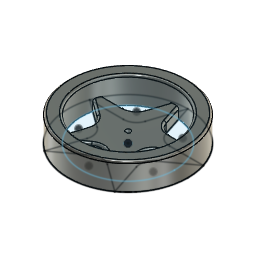
wheel (Autodesk Fusion 360 design; units mm, degrees)
Autodesk Fusion 360 part; units mm, degrees
note: some values were not read from the file. Set by a fixed rule: which sketch regions a step uses.
sketch "Esboço1" plane through (0, 0, 0) normal (0, 0, 1) x (1, 0, 0)
  circle A0 centre (0, 0) radius 45
  circle A1 centre (0, 0) radius 2
  circle A2 centre (0, 0) radius 35
  line L0 (-7.858, 20.8156) -> (0, 45)
  line L1 (-42.7975, 13.9058) -> (-17.3686, 13.9058)
  arc A3 (-17.3686, 13.9058) -> (-7.858, 20.8156) centre (-17.3686, 23.9058) ccw
  line L2 (0, 45) -> (7.858, 20.8156)
  line L3 (42.7975, 13.9058) -> (17.3686, 13.9058)
  arc A4 (7.858, 20.8156) -> (17.3686, 13.9058) centre (17.3686, 23.9058) ccw
  line L4 (-42.7975, 13.9058) -> (-22.2251, -1.041)
  line L5 (-26.4503, -36.4058) -> (-18.5923, -12.2214)
  arc A5 (-18.5923, -12.2214) -> (-22.2251, -1.041) centre (-28.1029, -9.1312) ccw
  line L6 (22.2251, -1.041) -> (42.7975, 13.9058)
  line L7 (26.4503, -36.4058) -> (18.5923, -12.2214)
  arc A6 (22.2251, -1.041) -> (18.5923, -12.2214) centre (28.1029, -9.1312) ccw
  line L8 (5.8779, -21.459) -> (26.4503, -36.4058)
  line L9 (-26.4503, -36.4058) -> (-5.8779, -21.459)
  arc A7 (5.8779, -21.459) -> (-5.8779, -21.459) centre (0, -29.5492) ccw
  line L10 (0, -1.5) -> (-1.3229, -1.5)
  line L11 (0, -1.5) -> (1.3229, -1.5)
  dimension "d1" = 10
  dimension "d2" = 10
  dimension "d3" = 10
  dimension "d4" = 10
  dimension "d5" = 10
  constraint coincident A0.centre A1.centre
  constraint concentric A0 A1
  constraint concentric A0 A2
  constraint coincident A0 L0.end
  constraint horizontal L1
  constraint coincident L3.start L1
  constraint coincident L5.start L0
  constraint tangent L1 A3
  constraint tangent L0 A3
  constraint coincident L7.start L2
  constraint coincident L1.start L3
  constraint tangent L2 A4
  constraint tangent L3 A4
  constraint coincident L7.start L4
  constraint coincident L0.end L5
  constraint tangent L4 A5
  constraint tangent L5 A5
  constraint coincident L5.start L6
  constraint coincident L0.end L7
  constraint tangent L6 A6
  constraint tangent L7 A6
  constraint coincident L3.start L9
  constraint coincident L1.start L8
  constraint tangent L9 A7
  constraint tangent L8 A7
  constraint coincident A1 L10.end
  constraint coincident A1 L11.end
  measures "d1" radius of A3
  measures "d2" radius of A4
  measures "d3" radius of A5
  measures "d4" radius of A6
  measures "d5" radius of A7
extrude "Extrusão1" add sketch "Esboço1" along normal blind 20 contours A0 A2 L6 L7 | A0 A2 L2 L3 | A2 L3 L6 | A2 L7 L8 | A0 A2 L8 L9 | A0 A2 L0 L1 | A2 L0 L2 | A0 A2 L4 L5 | A2 L5 L9 | A2 L1 L4
extrude "Extrusão2" add sketch "Esboço1" along normal blind 8 contours A2 L0 L1 A3 L2 L3 A4 L4 L5 A5 L6 L7 A6 L8 L9 A7 | A1 L10 L11 picked at (-0.096, -1.8264)
fillet "Arredondamento1" radius 1.5 17 edges at (-41.9547, -16.2727, 20) (-32.6315, 12.6565, 20) (-28.1917, 3.294, 8) (-18.5923, -6.041, 8) (-20.8714, -19.2356, 8) (-5.5789, 27.8298, 8) (-11.4907, 15.8156, 8) (-24.7438, 13.9058, 8) (24.7438, 13.9058, 8) (11.4907, 15.8156, 8) (5.5789, 27.8298, 8) (20.8714, -19.2356, 8) (18.5923, -6.041, 8) (28.1917, 3.294, 8) (-11.8445, -25.794, 8) (0, -19.5492, 8) (11.8445, -25.794, 8)
sketch "Esboço2" plane through (0, 0, 20) normal (0, 0, 1) x (-1, 0, 0)
  circle A0 centre (0, 0) radius 43.5
  circle A1 centre (0, 0) radius 36.5
